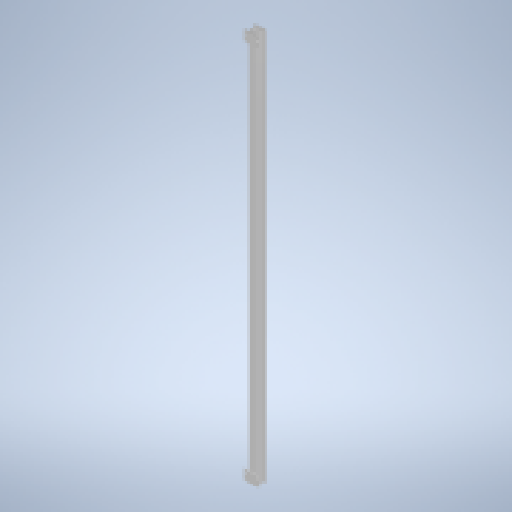
# Autodesk Inventor part: TrägerUI
Saved by Autodesk Inventor 2025 (Build 290162010, 162A)
## iProperties
Created: 2025-02-04
Part Number: TrägerUI
Material: Aluminium 6061, Katze
Document SubType Name: Modeling
Designer: Admin
Density: 2.7 g/cm^3
Appearance: Aluminium - flach(1)
Mass: 460.428 g
Surface Area: 1673.85 cm^2
Volume: 170.529 cm^3
Author: Admin
Autodesk Inventor part; units mm, degrees
ref_plane "YZ Plane" through (0, 0, 0) normal (1, 0, 0) x (0, 1, 0)
ref_plane "XZ Plane" through (0, 0, 0) normal (0, 1, 0) x (-1, 0, 0)
ref_plane "XY Plane" through (0, 0, 0) normal (0, 0, 1) x (1, 0, 0)
sketch "Skizze1" plane through (0, 0, 0) normal (0, 0, 1) x (1, 0, 0)
  line L0 (0, 0) -> (30, 0)
  line L1 (30, 0) -> (30, -2)
  line L2 (30, -2) -> (0, -2)
  line L3 (0, -2) -> (0, 0)
  line L4 (7.5, -2) -> (9.5, -2)
  line L5 (9.5, -2) -> (9.5, -22)
  line L6 (9.5, -22) -> (7.5, -22)
  line L7 (7.5, -22) -> (7.5, -2)
  line L8 (9.5, -22) -> (20.5, -22)
  line L9 (20.5, -22) -> (20.5, -20)
  line L10 (20.5, -20) -> (9.5, -20)
  line L11 (9.5, -20) -> (9.5, -22)
  line L12 (20.5, -22) -> (22.5, -22)
  line L13 (22.5, -22) -> (22.5, -2)
  line L14 (22.5, -2) -> (20.5, -2)
  line L15 (20.5, -2) -> (20.5, -22)
  line L16 (15, -20) -> (15, -2) construction
  point P0 (20.5, -2)
  point P1 (9.5, -2)
  dimension "d0" = 30
  dimension "d1" = 2
  dimension "d2" = 2
  dimension "d3" = 20
  dimension "d4" = 11
  dimension "d5" = 2
  dimension "d6" = 2
  dimension "d7" = 7.5
  dimension "d8" = 20.5
  dimension "d9" = 20
  dimension "d12" = 7.5
  constraints: 34 end point, 8 parallel, 4 horizontal, 4 perpendicular, 2 midpoint, 2 point on line, 1 vertical
  measures "d0" distance of L1.end L2.end
  measures "d1" distance of L0.end L1.end
  measures "d2" distance of L5.end L6.end
  measures "d3" distance of L4.end L5.end
  measures "d4" distance of L10.end L9.end
  measures "d5" distance of L9.end L8.end
  measures "d6" distance of L14.end L13.end
  measures "d7" distance from line of L2.end L7
  measures "d8" distance of L2.end L14.end
  measures "d9" vertical distance of L0.start L10.end
  measures "d12" distance from line of L13 L1.end
extrude "Extrusion1" add sketch "Skizze1" along normal blind 1000 contours L0 L1 L2 L3 | L2 L5 L6 L7 | L13 L12 L9 L15 L2 | L10 L9 L8 L5
sketch "Skizze2" plane through (22.5, -22, 0) normal (0, -1, 0) x (1, 0, 0)
  line L0 (7.5, 0) -> (7.5, 1000) projected
  line L1 (-26.5, 3) -> (11.5, 3)
  line L2 (11.5, 3) -> (11.5, 27)
  line L3 (-22.5, 0) -> (-22.5, 1000) projected
  line L4 (-26.5, 3) -> (-26.5, 27)
  line L5 (-26.5, 27) -> (11.5, 27)
  line L6 (-15, 0) -> (0, 0) projected
  line L7 (-26.5, 997) -> (11.5, 997)
  line L8 (11.5, 997) -> (11.5, 973)
  line L9 (11.5, 973) -> (-26.5, 973)
  line L10 (-26.5, 973) -> (-26.5, 997)
  line L11 (-15, 1000) -> (0, 1000) projected
  line L12 (0, 0) -> (0, 1000) projected
  line L13 (-15, 0) -> (-15, 1000) projected
  line L14 (-13, 0) -> (-13, 1000) projected
  point P0 (7.5, 3)
  point P1 (7.5, 27)
  dimension "d13" = 24
  dimension "d21" = 4
  dimension "d22" = 4
  dimension "d24" = 24
  dimension "d25" = 4
  dimension "d26" = 4
  dimension "d46" = 3
  dimension "d47" = 3
  constraints: 12 end point, 3 vertical, 1 horizontal, 1 parallel, 1 perpendicular, 6 other
  measures "d13" distance of L2.end L2.start
  measures "d21" distance from line of L2.start L0
  measures "d22" distance between parallel lines of L4 L3
  measures "d24" distance of L8.start L8.end
  measures "d25" distance between parallel lines of L10 L3
  measures "d26" distance between parallel lines of L0 L8
extrude "Extrusion2" add sketch "Skizze2" along normal blind 2 contours L1 L12 L5 L0 | L0 L5 L2 L1 | L1 L14 L5 L12 | L9 L12 L7 L0 | L0 L7 L8 L9 | L1 L13 L5 L14 | L9 L14 L7 L12 | L1 L3 L5 L13 | L9 L13 L7 L14 | L1 L4 L5 L3 | L9 L3 L7 L13 | L9 L10 L7 L3
sketch "Skizze3" plane through (22.5, -24, 0) normal (0, -1, 0) x (1, 0, 0)
  line L0 (-21, 18) -> (6, 18)
  line L1 (-22.5, 3) -> (11.5, 3) projected
  line L2 (-15, 997) -> (-15, 1000) projected
  line L3 (-15, 0) -> (-15, 1000) projected
  line L4 (0, 0) -> (0, 1000) projected
  line L5 (0, 0) -> (0, 3) projected
  line L6 (6, 985) -> (-21, 985)
  line L7 (0, 27) -> (0, 973) projected
  line L8 (0, 3) -> (0, 27) projected
  line L9 (-15, 0) -> (-15, 3) projected
  line L10 (-15, 27) -> (-15, 973) projected
  line L11 (0, 997) -> (0, 1000) projected
  line L12 (0, 973) -> (0, 997) projected
  line L13 (-15, 3) -> (-15, 27) projected
  line L14 (-15, 973) -> (-15, 997) projected
  point P0 (-22.5, 0)
  point P1 (11.5, 3)
  dimension "d17" = 15
  dimension "d19" = 6
  dimension "d23" = 15
  dimension "d27" = 6
  dimension "d28" = 6
  constraints: 4 end point, 1 horizontal, 1 perpendicular, 1 other
  measures "d19" distance from line of L4 L0.end
  measures "d23" distance from line of L2.end L6
  measures "d27" distance from line of L6.end L2
  measures "d28" distance from line of L4 L6.start
hole "Bohrung1" at (1.5, -24, 18) at (28.5, -24, 18) at (1.5, -24, 985) at (28.5, -24, 985) direction (0, 1, 0) diameter 5.5 depth 2 tip angle 118 clearance for "Flachkopfmaschinenschraube" size "M5" standard "ANSI Metrisches M Profil"
